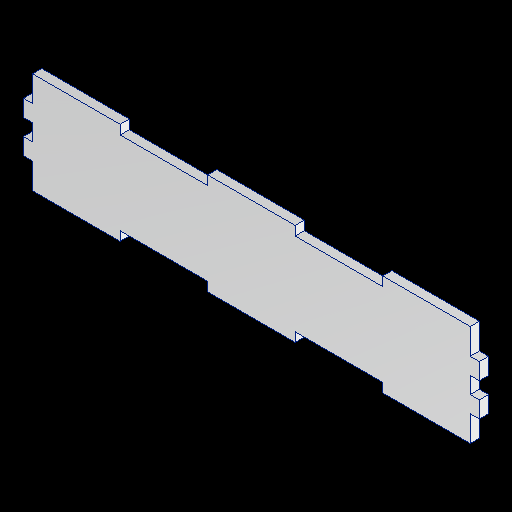
# Autodesk Inventor part: SideDriveArmorPlate
Saved by Autodesk Inventor 2022 (Build 260153000, 153)
## iProperties
Created: 2022-03-07
Part Number: SideDriveArmorPlate
Material: Aluminum 6061
Document SubType Name: Modeling
Designer: tandu
Density: 2.7 g/cm^3
Appearance: Aluminum - Flat
Mass: 2719.41 g
Surface Area: 1800.64 cm^2
Volume: 1007.19 cm^3
Thickness: 0.50000000 in
Author: tandu
Autodesk Inventor part; units mm, degrees
ref_plane "YZ Plane" through (0, 0, 0) normal (1, 0, 0) x (0, 1, 0)
ref_plane "XZ Plane" through (0, 0, 0) normal (0, 1, 0) x (-1, 0, 0)
ref_plane "Work Plane1" through (0, 0, 0) normal (0, 0, 1) x (1, 0, 0)
sketch "Sketch1" plane through (0, 0, 0) normal (0, 0, 1) x (1, 0, 0)
  line L0 (-25.4, 19.05) -> (-25.4, -584.2) construction
  line L1 (88.9, 19.0492) -> (88.9, -584.2008) construction
  line L2 (0, 19.05) -> (-25.4, 19.05) projected
  line L3 (-2.54, 19.05) -> (-2.54, 31.75) projected
  line L4 (-2.54, 31.75) -> (20.32, 31.75) projected
  line L5 (20.32, 19.05) -> (20.32, 31.75) projected
  line L6 (43.18, 19.05) -> (66.04, 19.05) construction
  line L7 (66.04, 19.05) -> (66.04, 31.75) projected
  line L8 (43.18, 31.75) -> (66.04, 31.75) projected
  line L9 (43.18, 19.05) -> (43.18, 31.75) projected
  line L10 (88.9, 19.0492) -> (63.5, 19.0492) projected
  line L11 (20.32, 19.05) -> (43.18, 19.05) projected
  line L12 (-2.54, -596.9) -> (20.32, -596.9) projected
  line L13 (20.32, -596.9) -> (20.32, -584.2) projected
  line L14 (-2.54, -584.2) -> (20.32, -584.2) construction
  line L15 (-2.54, -596.9) -> (-2.54, -584.2) projected
  line L16 (43.18, -596.9) -> (66.04, -596.9) projected
  line L17 (66.04, -596.9) -> (66.04, -584.2) projected
  line L18 (43.18, -584.2) -> (66.04, -584.2) construction
  line L19 (43.18, -596.9) -> (43.18, -584.2) projected
  line L20 (20.32, -584.2) -> (43.18, -584.2) projected
  line L21 (-2.54, -584.2) -> (-25.4, -584.2)
  line L22 (66.04, -584.2) -> (88.9, -584.2008)
  line L23 (-25.4, -584.2) -> (-38.1, -584.2)
  line L24 (-38.1, -584.2) -> (-38.1, -463.55)
  line L25 (-38.1, -463.55) -> (-25.4, -463.55)
  line L26 (-25.4, -463.55) -> (-25.4, -584.2) construction
  line L27 (-38.1, -463.55) -> (-25.4, -463.55)
  line L28 (-25.4, -463.55) -> (-25.4, -342.9)
  line L29 (-25.4, -342.9) -> (-38.1, -342.9)
  line L30 (-38.1, -342.9) -> (-38.1, -463.55) construction
  line L31 (-25.4, -342.9) -> (-38.1, -342.9)
  line L32 (-38.1, -342.9) -> (-38.1, -222.25)
  line L33 (-38.1, -222.25) -> (-25.4, -222.25)
  line L34 (-25.4, -222.25) -> (-25.4, -342.9) construction
  line L35 (-38.1, -222.25) -> (-25.4, -222.25)
  line L36 (-25.4, -222.25) -> (-25.4, -101.6)
  line L37 (-25.4, -101.6) -> (-38.1, -101.6)
  line L38 (-38.1, -101.6) -> (-38.1, -222.25) construction
  line L39 (-38.1, -101.6) -> (-25.4, -101.6)
  line L40 (-25.4, -101.6) -> (-25.4, 19.05) construction
  line L41 (-25.4, 19.05) -> (-38.1, 19.05)
  line L42 (-38.1, 19.05) -> (-38.1, -101.6)
  line L43 (31.75, -584.2) -> (31.75, 19.05) construction
  line L44 (88.9, -584.2) -> (101.6, -584.2)
  line L45 (101.6, -584.2) -> (101.6, -463.55)
  line L46 (101.6, -463.55) -> (88.9, -463.55)
  line L47 (88.9, -463.55) -> (88.9, -342.9)
  line L48 (88.9, -342.9) -> (101.6, -342.9)
  line L49 (101.6, -342.9) -> (101.6, -222.25)
  line L50 (101.6, -222.25) -> (88.9, -222.25)
  line L51 (88.9, -222.25) -> (88.9, -101.6)
  line L52 (88.9, -101.6) -> (101.6, -101.6)
  line L53 (88.9, 19.05) -> (101.6, 19.05)
  line L54 (101.6, 19.05) -> (101.6, -101.6)
  line L55 (66.04, -584.2) -> (66.04, -596.9)
  line L56 (43.18, -596.9) -> (66.04, -596.9)
  line L57 (-2.54, -584.2) -> (-2.54, -596.9)
  line L58 (-2.54, 19.05) -> (-25.4, 19.05)
  line L59 (66.04, 19.05) -> (88.9, 19.05)
  line L60 (-2.54, 19.05) -> (-2.54, 31.75)
  line L61 (66.04, 31.75) -> (66.04, 19.05)
  line L62 (101.6, 19.05) -> (66.04, 19.05)
  line L63 (66.04, 31.75) -> (43.18, 31.75)
  line L64 (43.18, 31.75) -> (43.18, 19.05)
  line L65 (20.32, 19.05) -> (43.18, 19.05)
  line L66 (20.32, 19.05) -> (20.32, 31.75)
  line L67 (-2.54, 31.75) -> (20.32, 31.75)
  line L68 (-2.54, -596.9) -> (20.32, -596.9)
  line L69 (20.32, -584.2) -> (20.32, -596.9)
  line L70 (20.32, -584.2) -> (43.18, -584.2)
  line L71 (43.18, -596.9) -> (43.18, -584.2)
  line L72 (-38.1, -463.55) -> (-25.4, -463.55)
  line L73 (101.6, -463.55) -> (88.9, -463.55)
  line L74 (101.6, -342.9) -> (88.9, -342.9)
  line L75 (101.6, -222.25) -> (88.9, -222.25)
  line L76 (-38.1, -584.2) -> (-2.54, -584.2)
  line L77 (66.04, -584.2) -> (101.6, -584.2)
  point P0 (0, 0)
  dimension "d0" = 12.7
  constraints: 114 end point, 21 collinear, 14 symmetric about line, 10 parallel, 9 perpendicular, 8 horizontal, 3 point on line, 2 midpoint
  measures "d0" distance of L0.start L41.end
extrude "Extrusion1" add sketch "Sketch1" along normal blind 12.7
equation "\"d1\" = Thickness"
equation "\"Thickness\" = 12.7"
body "Solid1"
